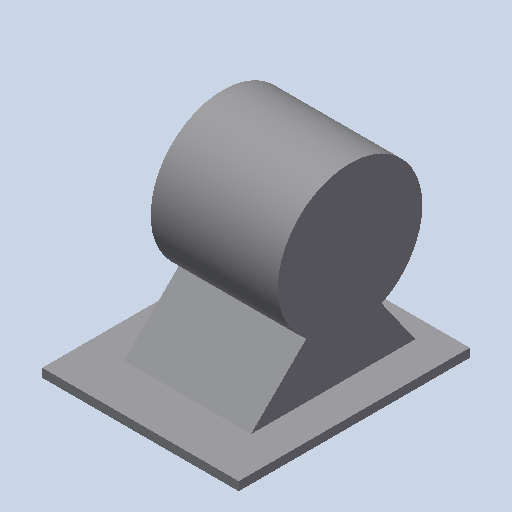
# Autodesk Inventor part: Rueda loca
Saved by Autodesk Inventor 2025 (Build 290162000, 162)
## iProperties
Created: 2024-10-07
Part Number: Rueda loca
Material: Generic
Document SubType Name: Modeling
Designer: feder
Density: 1 g/cm^3
Appearance: Default
Author: feder
Autodesk Inventor part; units mm, degrees
ref_plane "YZ Plane" through (0, 0, 0) normal (1, 0, 0) x (0, 1, 0)
ref_plane "XZ Plane" through (0, 0, 0) normal (0, 1, 0) x (-1, 0, 0)
ref_plane "XY Plane" through (0, 0, 0) normal (0, 0, 1) x (1, 0, 0)
sketch "Sketch1" plane through (0, 0, 0) normal (0, 1, 0) x (-1, 0, 0)
  line L0 (0, 0) -> (-34, 0)
  line L1 (-34, 0) -> (-34, -40)
  line L2 (-34, -40) -> (0, -40)
  line L3 (0, -40) -> (0, 0)
  dimension "d0" = 40
  dimension "d1" = 34
  constraints: 8 end point, 2 parallel, 1 horizontal, 1 perpendicular
  measures "d0" distance of L2.end L0.start
  measures "d1" distance of L1.end L2.end
extrude "Extrusion1" add sketch "Sketch1" along normal blind 1.5
sketch "Sketch2" plane through (34, 0, 0) normal (1, 0, 0) x (0, 0, -1)
  line L0 (0, 1.5) -> (40, 1.5) projected
  line L1 (8.1604, 1.5) -> (27.7337, 21)
  line L2 (27.7337, 21) -> (22.8205, 21)
  line L3 (22.8205, 21) -> (36.5617, 1.5)
  circle A0 centre (25.2771, 21) radius 12.5
  line L4 (0, 0) -> (40, 0) projected
  point P0 (17.731, 11.0347)
  point P1 (30.7424, 9.7581)
  dimension "d4" = 25
  dimension "d5" = 21
  constraints: 6 end point, 2 point on line, 1 centre point, 1 midpoint, 1 parallel
  measures "d4" diameter of A0
  measures "d5" distance from line of L4 A0.centre
extrude "Extrusion2" add sketch "Sketch2" against normal up to surface (34 mm away) contours L1 A0 L3 L0 | L3 L2 L1 | A0 L3 L1 | L1 L3 A0
sketch "Sketch3" plane through (34, 0, -40) normal (0, 0, -1) x (-1, 0, 0)
  line L0 (34, 1.5) -> (0, 1.5) projected
  line L1 (0, 33.5) -> (34, 33.5) projected
  line L2 (0, 1.5) -> (6, 1.5)
  line L3 (6, 1.5) -> (6, 33.5)
  line L4 (6, 33.5) -> (0, 33.5)
  line L5 (0, 33.5) -> (0, 1.5)
  line L6 (34, 33.5) -> (28, 33.5)
  line L7 (28, 33.5) -> (28, 1.5)
  line L8 (28, 1.5) -> (34, 1.5)
  line L9 (34, 1.5) -> (34, 33.5)
  point P0 (34, 0)
  point P1 (28, 1.5)
  dimension "d8" = 6
  dimension "d9" = 6
  constraints: 16 end point, 4 parallel, 3 point on line, 2 horizontal, 2 perpendicular
  measures "d8" distance of L4.end L3.end
  measures "d9" distance of L8.end L7.end
extrude "Extrusion3" cut sketch "Sketch3" against normal through all contours L0 L7 L1 L9 | L0 L5 L1 L3
body "Solid1"
